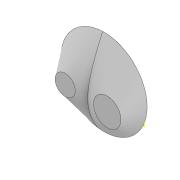
# Autodesk Inventor part: Radius_1
Saved by Autodesk Inventor 2020 (Build 240168000, 168)
## iProperties
Created: 2021-01-23
Part Number: Radius_1
Material: Generic
Document SubType Name: Modeling
Designer: deox
Density: 1 g/cm^3
Appearance: Default
Author: deox
Autodesk Inventor part; units mm, degrees
ref_plane "YZ Plane" through (0, 0, 0) normal (1, 0, 0) x (0, 1, 0)
ref_plane "XZ Plane" through (0, 0, 0) normal (0, 1, 0) x (-1, 0, 0)
sketch "Sketch1" plane through (0, 0, 0) normal (0, 0, 1) x (1, 0, 0)
  circle A0 centre (-6.1857, 1.9585) radius 3.3651
  point P0 (0, 0)
  constraints: 1 centre point
ref_plane "Work Plane1" through (0, 0, -6.75) normal (0, 0, 1) x (1, 0, 0)
sketch "Sketch2" plane through (0, 0, -6.75) normal (0, 0, 1) x (1, 0, 0)
  circle A0 centre (0, 2.5402) radius 14.366
  point P0 (0, 0)
  constraints: 1 centre point
sketch "Sketch3" plane through (0, 0, 0) normal (0, 0, 1) x (1, 0, 0)
  circle A0 centre (7.8146, 1.1828) radius 4.5733 projected
  point P0 (0, 0)
loft "Loft1" add profiles "Sketch2", "Sketch1"
loft "Loft2" add profiles "Sketch3" section 1 edges at (-14.366, 2.5402, -6.75)
body "Solid1"
